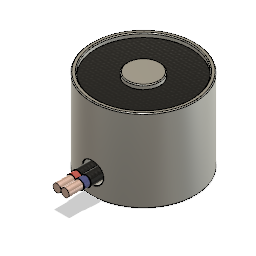
20 (Autodesk Fusion 360 design; units mm, degrees)
Autodesk Fusion 360 part; units mm, degrees
sketch "Sketch1" plane through (0, 0, 0) normal (0, 1, 0) x (1, 0, 0)
  circle A0 centre (0, 0) radius 12.5
  dimension "d1" = 25
  constraint coincident A0.centre origin
  measures "d1" diameter of A0
extrude "Extrude1" add sketch "Sketch1" along normal blind 20
sketch "Sketch2" plane through (0, 20, 0) normal (0, 1, 0) x (-1, 0, 0)
  circle A0 centre (0, 0) radius 12.5
  circle A1 centre (0, 0) radius 4
  circle A2 centre (0, 0) radius 11.5
  dimension "d4" = 8
  dimension "d5" = 23
  constraint coincident A0.centre A1.centre
  measures "d4" diameter of A1
  measures "d5" diameter of A2
extrude "Extrude2" cut sketch "Sketch2" against normal blind 1 contours A2
fillet "Fillet1" radius 0.2 4 edges at (3.7293, 20, -1.4465) (10.7218, 20, 4.1586) (-11.6541, 20, 4.5202) (-11.6541, 0, 4.5202)
sketch "Sketch3" plane through (0, 0, 0) normal (0, 0, 1) x (1, 0, 0)
  circle A0 centre (0, 5) radius 2.5
  dimension "d10" = 5
  dimension "d11" = 5
  constraint vertical origin A0.centre
  measures "d10" diameter of A0
  measures "d11" distance of origin A0.centre
extrude "Extrude3" cut sketch "Sketch3" along normal blind 22
fillet "Fillet2" radius 0.1 1 edges at (-2.5, 5, 12.2474)
sketch "Sketch4" plane through (0, 0, 0) normal (0, 0, 1) x (1, 0, 0)
  circle A0 centre (0, 5) radius 2.5
  line L0 (-0.134, 5.5) -> (0.134, 5.5)
  line L1 (-0.134, 4.5) -> (0.134, 4.5)
  arc A1 (-0.134, 5.5) -> (-0.134, 4.5) centre (-1, 5) ccw
  arc A2 (0.134, 4.5) -> (0.134, 5.5) centre (1, 5) ccw
  arc A3 (0, 4.1693) -> (0, 5.8307) centre (1, 5) ccw
  arc A4 (0, 5.8307) -> (0, 4.1693) centre (-1, 5) ccw
  dimension "d16" = 2
  dimension "d17" = 2
  dimension "d18" = 5
  dimension "d19" = 1
  dimension "d20" = 0.5
  dimension "d21" = 0.5
  dimension "d22" = 0.5
  dimension "d23" = 0.3
  constraint tangent A1 A2
  constraint horizontal L0
  measures "d16" diameter of A1
  measures "d17" diameter of A2
  measures "d18" vertical distance of origin A2.centre
  measures "d19" horizontal distance of origin A1.centre
  measures "d20" distance of A1.centre L0
  measures "d21" distance of A2.centre L1
  measures "d22" distance of A1.centre L1
extrude "Extrude4" add sketch "Sketch4" along normal blind 20 contours L0 L1 A1 A2
extrude "Extrude5" add sketch "Sketch4" along normal blind 15 contours A3 A4
sketch "Sketch5" plane through (0, 0, 20) normal (0, 0, 1) x (1, 0, 0)
  arc A0 (-0.134, 5.5) -> (-0.134, 4.5) centre (-1, 5) ccw
  line L0 (-0.134, 4.5) -> (0.134, 4.5)
  arc A1 (0.134, 4.5) -> (0.134, 5.5) centre (1, 5) ccw
  line L1 (0.134, 5.5) -> (-0.134, 5.5)
  circle A2 centre (1, 5) radius 1
  circle A3 centre (-1, 5) radius 1
  constraint concentric A1 A2
  constraint concentric A0 A3
extrude "Extrude6" cut sketch "Sketch5" against normal blind 5 contours L1 A2 A3 | L0 A2 A3
sketch "Sketch6" plane through (0, 0, 15) normal (0, 0, 1) x (1, 0, 0)
  circle A0 centre (-1, 5) radius 1
  circle A1 centre (1, 5) radius 1
  arc A2 (0, 5.8307) -> (0, 4.1693) centre (-1, 5) ccw
  arc A3 (0, 4.1693) -> (0, 5.8307) centre (1, 5) ccw
  arc A4 (0, 4.4321) -> (0, 5.5679) centre (1, 5) ccw
  arc A5 (0, 5.5679) -> (0, 4.4321) centre (-1, 5) ccw
  circle A6 centre (-1, 5) radius 1
  dimension "d30" = -0.15
extrude "Extrude7" add sketch "Sketch6" along normal blind 1.5 contours A4 A5
